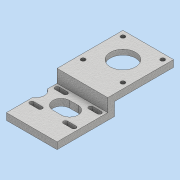
# Autodesk Inventor part: Uchwyt silnika krokowego osi X
Saved by Autodesk Inventor 2018 (Build 220112000, 112)
## iProperties
Created: 2019-01-25
Part Number: Uchwyt silnika krokowego osi X
Material: Ogólny
Document SubType Name: Modeling
Designer: Dawid
Density: 1 g/cm^3
Appearance: Aluminium odlewane
Author: Dawid
Autodesk Inventor part; units mm, degrees
ref_plane "YZ Plane" through (0, 0, 0) normal (1, 0, 0) x (0, 1, 0)
ref_plane "XZ Plane" through (0, 0, 0) normal (0, 1, 0) x (-1, 0, 0)
ref_plane "XY Plane" through (0, 0, 0) normal (0, 0, 1) x (1, 0, 0)
sketch "Szkic1" plane through (0, 0, 0) normal (0, 0, 1) x (1, 0, 0)
  line L0 (-30, -35) -> (30, -35)
  line L1 (30, -35) -> (30, 35)
  line L2 (30, 35) -> (-30, 35)
  line L3 (-30, 35) -> (-30, -35)
  line L4 (-30, -35) -> (30, 35) construction
  line L5 (30, -35) -> (-30, 35) construction
  point P0 (0, 0)
  dimension "d0" = 60
  dimension "d1" = 70
  constraints: 12 end point, 2 midpoint, 2 parallel, 1 horizontal, 1 perpendicular
  measures "d0" distance of L2.end L1.end
  measures "d1" distance of L1.end L0.end
extrude "Wyciągnięcie proste1" add sketch "Szkic1" along normal blind 8
sketch "Szkic2" plane through (0, 0, 0) normal (0, 0, -1) x (-1, 0, 0)
  line L0 (30, -35) -> (-30, -35) projected
  line L1 (30, 35) -> (30, -35) projected
  line L2 (-30, 35) -> (30, 35) projected
  line L3 (-30, -35) -> (-30, 35) projected
  line L4 (23.57, 5) -> (23.57, 28.57)
  line L5 (23.57, 28.57) -> (-23.57, 28.57)
  line L6 (-23.57, 28.57) -> (-23.57, -18.57)
  line L7 (-23.57, -18.57) -> (23.57, -18.57)
  line L8 (23.57, -18.57) -> (23.57, 5)
  circle A0 centre (23.57, 28.57) radius 2.5
  circle A1 centre (-23.57, 28.57) radius 2.5
  circle A2 centre (-23.57, -18.57) radius 2.5
  circle A3 centre (23.57, -18.57) radius 2.5
  line L9 (0, 0) -> (0, 5)
  dimension "d6" = 47.14
  dimension "d7" = 47.14
  dimension "d8" = 47.14
  dimension "d9" = 5
  dimension "d10" = 5
  dimension "d11" = 5
  dimension "d12" = 5
  dimension "d15" = 5
  constraints: 12 end point, 4 centre point, 4 coincident, 2 perpendicular, 1 point on line, 1 vertical
  measures "d6" distance of L4.end L5.end
  measures "d7" distance of L5.end L6.end
  measures "d8" distance of L6.end L7.end
  measures "d9" diameter of A0
  measures "d10" diameter of A1
  measures "d11" diameter of A2
  measures "d12" diameter of A3
  measures "d15" distance of L9.start L9.end
extrude "Wyciągnięcie proste3" cut sketch "Szkic2" against normal up to next contours A0 L5 L4 | L4 L5 A0 | A3 L7 L8 | L8 L7 A3 | A1 L6 L5 | L5 L6 A1 | A2 L6 L7 | L7 L6 A2
sketch "Szkic4" plane through (0, 0, 8) normal (0, 0, 1) x (1, 0, 0)
  line L0 (-30, -35) -> (30, -35) projected
  line L1 (30, -35) -> (30, -43)
  line L2 (30, -43) -> (-30, -43)
  line L3 (-30, -43) -> (-30, -35)
  point P0 (0, 0)
  dimension "d18" = 8
  constraints: 6 end point, 2 perpendicular, 1 vertical
  measures "d18" distance of L0.end L1.end
extrude "Wyciągnięcie proste4" add sketch "Szkic4" against normal blind 43.4
sketch "Szkic5" plane through (0, 0, 8) normal (0, 0, 1) x (1, 0, 0)
  circle A0 centre (-23.57, -18.57) radius 2.5 projected
  circle A1 centre (23.57, 28.57) radius 2.5 projected
  circle A2 centre (-23.57, 28.57) radius 2.5 projected
  circle A3 centre (23.57, -18.57) radius 2.5 projected
  line L0 (30, 35) -> (30, -43) projected
  line L1 (30, 35) -> (-30, 35) projected
  line L2 (-30, 35) -> (-30, -43) projected
  line L3 (30, -43) -> (-30, -43) projected
  line L4 (23.57, -18.57) -> (-23.57, 28.57)
  line L5 (-23.57, -18.57) -> (23.57, 28.57)
  circle A4 centre (0, 5) radius 15
  point P0 (0, 0)
  dimension "d21" = 30
  constraints: 4 end point, 1 centre point, 1 midpoint
  measures "d21" diameter of A4
extrude "Wyciągnięcie proste5" cut sketch "Szkic5" against normal up to next contours A4 L4 L5 | L5 L4 A4 | L5 A4 L4 | L4 A4 L5
thread "Gwint1" size "M5x0.8" class "6H" standard "ANSI Metric M Profile" full length
thread "Gwint2" size "M5x0.8" class "6H" standard "ANSI Metric M Profile" full length
thread "Gwint3" size "M5x0.8" class "6H" standard "ANSI Metric M Profile" full length
thread "Gwint4" size "M5x0.8" class "6H" standard "ANSI Metric M Profile" full length
sketch "Szkic10" plane through (0, 0, 0) normal (0, 0, -1) x (-1, 0, 0)
  circle A0 centre (0, 5) radius 15 projected
  circle A1 centre (0, 5) radius 19.5
  point P0 (0, 0)
  dimension "d59" = 39
  constraints: 1 centre point, 1 coincident
  measures "d59" diameter of A1
extrude "Wyciągnięcie proste10" cut sketch "Szkic10" against normal blind 2
sketch "Szkic12" plane through (0, 0, -35.4) normal (0, 0, -1) x (-1, 0, 0)
  line L0 (30, -35) -> (-30, -35) projected
  line L1 (-30, -35) -> (-30, -43) projected
  line L2 (-30, -43) -> (30, -43) projected
  line L3 (30, -43) -> (30, -35) projected
  point P0 (0, 0)
extrude "Wyciągnięcie proste12" cut sketch "Szkic12" against normal blind 20
sketch "Szkic13" plane through (-30, -43, 8) normal (0, -1, 0) x (1, 0, 0)
  line L0 (0, -23.4) -> (60, -23.4) projected
  line L1 (0, 0) -> (0, -23.4) projected
  line L2 (60, 0) -> (60, -23.4) projected
  line L3 (60, -23.4) -> (60, -15.4)
  line L4 (60, -8) -> (60, -23.4) projected
  line L5 (60, -15.4) -> (0, -15.4)
  point P0 (30, -8)
  dimension "d66" = 8
  constraints: 4 end point, 2 point on line, 1 perpendicular
  measures "d66" distance of L0.end L3.end
extrude "Wyciągnięcie proste13" add sketch "Szkic13" along normal blind 60
sketch "Szkic16" plane through (-30, -43, -7.4) normal (0, 0, 1) x (1, 0, 0)
  line L0 (60, -60) -> (0, -60)
  line L1 (60, 0) -> (60, -60)
  line L2 (0, 0) -> (60, 0)
  line L3 (0, 0) -> (0, -60)
  circle A0 centre (30, -20) radius 6.5
  line L4 (30, -20) -> (35, -20)
  line L5 (30, -20) -> (25, -20)
  arc A1 (35, -30) -> (35, -10) centre (35, -20) ccw
  arc A2 (25, -10) -> (25, -30) centre (25, -20) ccw
  line L6 (25, -10) -> (35, -10)
  line L7 (35, -30) -> (25, -30)
  point P0 (30, 43)
  dimension "d87" = 5
  dimension "d88" = 5
  dimension "d89" = 10
  constraints: 16 end point, 4 point on circle, 3 centre point, 3 horizontal, 2 coincident, 1 parallel
  measures "d87" distance of L4.start L4.end
  measures "d88" distance of L4.start L5.end
  measures "d89" radius of A1
extrude "Wyciągnięcie proste15" cut sketch "Szkic16" against normal up to next contours A0 | L7 A2 L6 A1
sketch "Szkic17" plane through (-30, -43, -7.4) normal (0, 0, 1) x (1, 0, 0)
  line L0 (25, -10) -> (35, -10) projected
  arc A0 (35, -30) -> (35, -10) centre (35, -20) ccw projected
  line L1 (35, -30) -> (25, -30) projected
  arc A1 (25, -10) -> (25, -30) centre (25, -20) ccw projected
  line L2 (0, 0) -> (60, 0) projected
  line L3 (0, 0) -> (0, -60) projected
  line L4 (60, -60) -> (0, -60) projected
  line L5 (60, 0) -> (60, -60) projected
  line L6 (60, 0) -> (60, -5)
  line L7 (60, 8) -> (60, -60) projected
  line L8 (30, -30) -> (30, -35)
  line L9 (60, -5) -> (57.5, -5)
  arc A2 (55, -7.5) -> (55, -2.5) centre (55, -5) ccw
  arc A3 (45, -2.5) -> (45, -7.5) centre (45, -5) ccw
  line L10 (55, -7.5) -> (45, -7.5)
  line L11 (60, -5) -> (57.5, -5)
  line L12 (55, -2.5) -> (45, -2.5)
  line L13 (60, -35) -> (57.5, -35)
  arc A4 (55, -37.5) -> (55, -32.5) centre (55, -35) ccw
  arc A5 (45, -32.5) -> (45, -37.5) centre (45, -35) ccw
  line L14 (55, -37.5) -> (45, -37.5)
  line L15 (55, -32.5) -> (45, -32.5)
  line L16 (30, -35) -> (42.5, -35)
  line L17 (57.5, -35) -> (60, -35)
  line L18 (0, -5) -> (2.5, -5)
  line L19 (0, -35) -> (2.5, -35)
  arc A6 (15, -7.5) -> (15, -2.5) centre (15, -5) ccw
  line L20 (15, -7.5) -> (5, -7.5)
  line L21 (15, -2.5) -> (5, -2.5)
  arc A7 (5, -2.5) -> (5, -7.5) centre (5, -5) ccw
  arc A8 (15, -37.5) -> (15, -32.5) centre (15, -35) ccw
  line L22 (15, -37.5) -> (5, -37.5)
  line L23 (15, -32.5) -> (5, -32.5)
  arc A9 (5, -32.5) -> (5, -37.5) centre (5, -35) ccw
  line L24 (42.5, -5) -> (17.5, -5)
  line L25 (2.5, -5) -> (0, -5)
  line L26 (30, -35) -> (17.5, -35)
  line L27 (2.5, -35) -> (0, -35)
  point P0 (30, 43)
  dimension "d92" = 5
  dimension "d93" = 5
  dimension "d98" = 2.5
  dimension "d99" = 2.5
  dimension "d100" = 2.5
  dimension "d101" = 2.5
  constraints: 42 end point, 24 point on circle, 8 centre point, 5 perpendicular, 4 horizontal, 4 point on line, 1 midpoint, 1 vertical
  measures "d92" distance of L2.end L6.end
  measures "d93" distance of L8.start L8.end
  measures "d98" distance of L6.end L9.end
  measures "d99" distance of L13.end L13.start
  measures "d100" distance of L18.end L18.start
  measures "d101" distance of L19.end L19.start
extrude "Wyciągnięcie proste16" cut sketch "Szkic17" against normal up to next contours A5 L15 A4 L14 | A8 L22 A9 L23 | A2 L10 A3 L12 | A7 L21 A6 L20
sketch "Szkic18" plane through (-30, -43, -7.4) normal (0, 0, 1) x (1, 0, 0)
  line L0 (55, -5) -> (50, -5)
  line L1 (55, -35) -> (50, -35)
  line L2 (5, -5) -> (10, -5)
  line L3 (5, -35) -> (10, -35)
  circle A0 centre (10, -5) radius 2
  circle A1 centre (10, -35) radius 2
  circle A2 centre (50, -35) radius 2
  circle A3 centre (50, -5) radius 2
  line L4 (45, -2.5) -> (55, -2.5) projected
  arc A4 (55, -7.5) -> (55, -2.5) centre (55, -5) ccw projected
  line L5 (55, -7.5) -> (45, -7.5) projected
  arc A5 (45, -2.5) -> (45, -7.5) centre (45, -5) ccw projected
  line L6 (15, -37.5) -> (5, -37.5) projected
  arc A6 (5, -32.5) -> (5, -37.5) centre (5, -35) ccw projected
  line L7 (5, -32.5) -> (15, -32.5) projected
  arc A7 (15, -37.5) -> (15, -32.5) centre (15, -35) ccw projected
  line L8 (5, -2.5) -> (15, -2.5) projected
  arc A8 (15, -7.5) -> (15, -2.5) centre (15, -5) ccw projected
  line L9 (15, -7.5) -> (5, -7.5) projected
  arc A9 (5, -2.5) -> (5, -7.5) centre (5, -5) ccw projected
  line L10 (55, -37.5) -> (45, -37.5) projected
  arc A10 (45, -32.5) -> (45, -37.5) centre (45, -35) ccw projected
  line L11 (45, -32.5) -> (55, -32.5) projected
  arc A11 (55, -37.5) -> (55, -32.5) centre (55, -35) ccw projected
  line L12 (25, -10) -> (35, -10) projected
  arc A12 (35, -30) -> (35, -10) centre (35, -20) ccw projected
  line L13 (35, -30) -> (25, -30) projected
  arc A13 (25, -10) -> (25, -30) centre (25, -20) ccw projected
  line L14 (0, 0) -> (60, 0) projected
  line L15 (0, 0) -> (0, -60) projected
  line L16 (60, -60) -> (0, -60) projected
  line L17 (60, 0) -> (60, -60) projected
  line L18 (55, -5) -> (60, -5)
  line L19 (55, -35) -> (60, -35)
  line L20 (5, -5) -> (0, -5)
  line L21 (5, -35) -> (0, -35)
  point P0 (30, 43)
  dimension "d104" = 5
  dimension "d105" = 5
  dimension "d106" = 5
  dimension "d107" = 5
  dimension "d108" = 4
  dimension "d109" = 4
  dimension "d110" = 4
  dimension "d111" = 4
  constraints: 16 end point, 5 point on line, 4 centre point, 4 coincident, 4 horizontal, 3 perpendicular
  measures "d104" distance of L0.start L0.end
  measures "d105" distance of L1.start L1.end
  measures "d106" distance of L2.start L2.end
  measures "d107" distance of L3.start L3.end
  measures "d108" diameter of A0
  measures "d109" diameter of A1
  measures "d110" diameter of A2
  measures "d111" diameter of A3
sketch "Szkic19" plane through (-30, -43, -7.4) normal (0, 0, 1) x (1, 0, 0)
  line L0 (45, -2.5) -> (55, -2.5)
  arc A0 (55, -7.5) -> (55, -2.5) centre (55, -5) ccw
  line L1 (55, -7.5) -> (45, -7.5)
  arc A1 (45, -2.5) -> (45, -7.5) centre (45, -5) ccw
  line L2 (15, -37.5) -> (5, -37.5)
  arc A2 (5, -32.5) -> (5, -37.5) centre (5, -35) ccw
  line L3 (5, -32.5) -> (15, -32.5)
  arc A3 (15, -37.5) -> (15, -32.5) centre (15, -35) ccw
  line L4 (5, -2.5) -> (15, -2.5)
  arc A4 (15, -7.5) -> (15, -2.5) centre (15, -5) ccw
  line L5 (15, -7.5) -> (5, -7.5)
  arc A5 (5, -2.5) -> (5, -7.5) centre (5, -5) ccw
  line L6 (55, -37.5) -> (45, -37.5)
  arc A6 (45, -32.5) -> (45, -37.5) centre (45, -35) ccw
  line L7 (45, -32.5) -> (55, -32.5)
  arc A7 (55, -37.5) -> (55, -32.5) centre (55, -35) ccw
  line L8 (25, -10) -> (35, -10)
  arc A8 (35, -30) -> (35, -10) centre (35, -20) ccw
  line L9 (35, -30) -> (25, -30)
  arc A9 (25, -10) -> (25, -30) centre (25, -20) ccw
  line L10 (0, 0) -> (60, 0)
  line L11 (60, -60) -> (0, -60)
  line L12 (60, 0) -> (60, -60)
  line L13 (60, 0) -> (60, -60)
  line L14 (60, -60) -> (0, -60)
  line L15 (0, 0) -> (60, 0)
  circle A10 centre (29.9999, -20) radius 6.5
  circle A11 centre (-10.0001, -20) radius 6.5
  line L16 (-10.0001, -20) -> (-5.0001, -20)
  arc A12 (0, -28.6602) -> (0, -11.3398) centre (-5.0001, -20) ccw
  line L17 (0, 0) -> (0, -2.5)
  line L18 (0, -37.5) -> (0, -60)
  line L19 (0, -11.3398) -> (0, -2.5)
  line L20 (0, 8) -> (0, -60) projected
  line L21 (0, -28.6602) -> (0, -37.5)
  line L22 (-5.0001, -20) -> (-3.5001, -20)
  line L23 (0, -11.3398) -> (-3.5001, -11.3398)
  line L24 (-3.5001, -11.3398) -> (-3.5001, -28.6602)
  line L25 (-3.5001, -28.6602) -> (0, -28.6602)
  point P0 (30, 43)
  dimension "d112" = 13
  dimension "d113" = 13
  dimension "d114" = 4.9999
  dimension "d115" = 5
  constraints: 50 end point, 22 centre point, 22 point on circle, 2 perpendicular, 2 point on line, 1 coincident, 1 collinear, 1 horizontal, 1 midpoint, 1 vertical, 1 other
  measures "d112" diameter of A10
  measures "d113" diameter of A11
  measures "d114" distance of A10.centre A9.centre
  measures "d115" distance of L16.start L16.end
extrude "Wyciągnięcie proste17" cut sketch "Szkic19" against normal up to next contours A12 L20 | L20 L25 L24 L23
